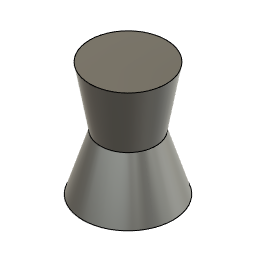
forme2 v1 (Autodesk Fusion 360 design; units mm, degrees)
Autodesk Fusion 360 part; units mm, degrees
sketch "Esquisse1" plane through (0, 0, 0) normal (0, 0, 1) x (1, 0, 0)
  line L0 (0, 0) -> (-65, 0)
  line L1 (-65, 0) -> (-40, 80)
  line L2 (-40, 80) -> (-55, 165)
  line L3 (-55, 165) -> (0, 165)
  line L4 (0, 165) -> (0, 0)
  dimension "d1" = 65
  dimension "d2" = 80
  dimension "d3" = 85
  dimension "d4" = 40
  dimension "d5" = 55
  constraint coincident L0.start L4.end
  constraint horizontal L0
  constraint horizontal L3
  constraint perpendicular L0 L4
  measures "d1" distance of L0.start L0.end
  measures "d2" vertical distance of L0.end L1.end
  measures "d3" vertical distance of L1.end L2.end
  measures "d4" distance of L1.end L4
  measures "d5" distance of L2.end L3.end
revolve "Révolution1" add sketch "Esquisse1" angle 360 about axis through (0, 165, 0) along (0, -1, 0)
shell "Coque1" thickness 2 removed faces 1 at (20.2416, 0, -0.2148)
